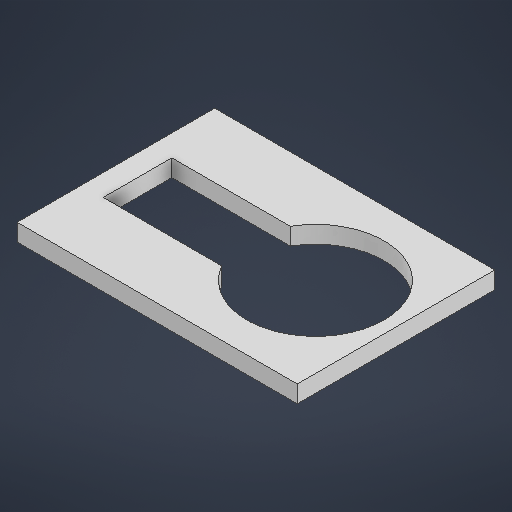
# Autodesk Inventor part: t1
Saved by Autodesk Inventor 2026 (Build 300175000, 175)
## iProperties
Created: 2025-04-19
Part Number: t1
Material: Generic
Document SubType Name: Modeling
Designer: ct_vi
Density: 1 g/cm^3
Appearance: Default
Author: ct_vi
Autodesk Inventor part; units mm, degrees
ref_plane "YZ Plane" through (0, 0, 0) normal (1, 0, 0) x (0, 1, 0)
ref_plane "XZ Plane" through (0, 0, 0) normal (0, 1, 0) x (-1, 0, 0)
ref_plane "XY Plane" through (0, 0, 0) normal (0, 0, 1) x (1, 0, 0)
sketch "Sketch1" plane through (0, 0, 0) normal (0, 1, 0) x (-1, 0, 0)
  line L0 (4.0829, 2.8794) -> (-4.0829, 2.8794)
  line L1 (-4.0829, 2.8794) -> (-4.0829, -2.8794)
  line L2 (-4.0829, -2.8794) -> (4.0829, -2.8794)
  line L3 (4.0829, -2.8794) -> (4.0829, 2.8794)
  line L4 (4.0829, 2.8794) -> (-4.0829, -2.8794) construction
  line L5 (-4.0829, 2.8794) -> (4.0829, -2.8794) construction
  line L6 (0, -1.0009) -> (3.455, -1.0009)
  line L7 (3.455, -1.0009) -> (3.455, 0.9991)
  line L8 (3.455, 0.9991) -> (0, 0.9991)
  line L9 (0, 0) -> (0, -1.0009)
  arc A0 (0.26, -0.1834) -> (0.26, 0.1834) centre (-1.7315, 0) ccw
  arc A1 (0.001, 0.9991) -> (0, -1.0009) centre (-1.7315, 0) ccw
  point P0 (0, 0)
  dimension "d1" = 2
  constraints: 20 end point, 4 parallel, 4 point on circle, 3 midpoint, 3 point on line, 2 centre point, 2 horizontal, 2 perpendicular
  measures "d1" distance of L7.end L6.end
extrude "Extrusion1" add sketch "Sketch1" along normal blind 0.5
body "Solid1"
